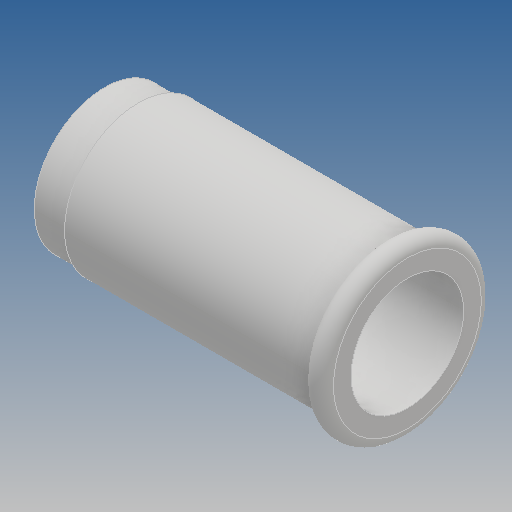
# Autodesk Inventor part: Zylinder
Saved by Autodesk Inventor 2018 (Build 220112000, 112)
## iProperties
Created: 2018-09-25
Part Number: Zylinder
Material: Generisch
Document SubType Name: Modeling
Designer: M.Knabel
Density: 1 g/cm^3
Appearance: Vorgabe
Mass: 6.34058 g
Surface Area: 54.1504 cm^2
Volume: 6.34058 cm^3
Author: M.Knabel
Autodesk Inventor part; units mm, degrees
ref_plane "YZ Plane" through (0, 0, 0) normal (1, 0, 0) x (0, 1, 0)
ref_plane "XZ Plane" through (0, 0, 0) normal (0, 1, 0) x (-1, 0, 0)
ref_plane "XY Plane" through (0, 0, 0) normal (0, 0, 1) x (1, 0, 0)
sketch "Skizze1" plane through (0, 0, 0) normal (0, 0, 1) x (1, 0, 0)
  line L0 (0, -2.4) -> (0, 14.4) projected
  line L1 (-30.1, 0) -> (30.1, 0) projected
  arc A0 (21.5, 10.5) -> (18.5, 10.5) centre (20, 10.5) ccw
  line L2 (21.5, 10.5) -> (21.5, 8)
  line L3 (21.5, 8) -> (-21.5, 8)
  line L4 (-21.5, 8) -> (-21.5, 10)
  line L5 (-21.5, 10) -> (-16.7, 10)
  line L6 (-16.7, 10) -> (-16.7, 10.5)
  line L7 (-16.7, 10.5) -> (18.5, 10.5)
  point P0 (0, 0)
  dimension "d0" = 3
  dimension "d1" = 21
  dimension "d2" = 16
  dimension "d3" = 43
  dimension "d4" = 4.8
  dimension "d5" = 20
  constraints: 12 end point, 6 perpendicular, 2 point on circle, 1 centre point, 1 point on line, 1 tangent, 1 other
  measures "d0" diameter of A0
  measures "d1" diameter of L7.end L1
  measures "d2" diameter of L3 L1
  measures "d3" distance between parallel lines of L4 L2
  measures "d4" distance from line of L5.end L4
  measures "d5" diameter of L5 L1
revolve "Umdrehung1" add sketch "Skizze1" angle 360 about axis through (-10, 0, 0) along (1, 0, 0)
